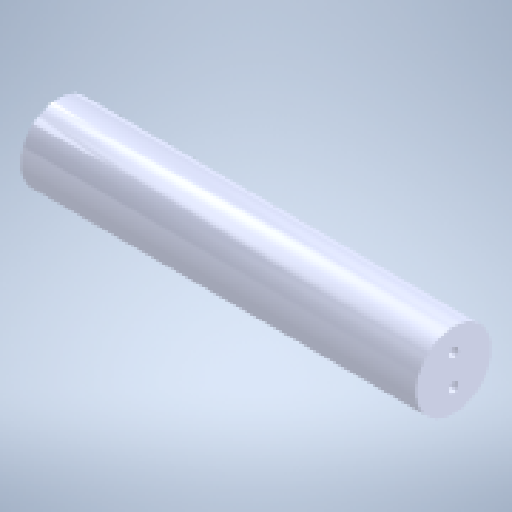
# Autodesk Inventor part: Herramienta Marcador Tubo
Saved by Autodesk Inventor 2023 (Build 270158000, 158)
## iProperties
Created: 2009-11-11
Part Number: Herramienta Marcador Tubo
Material: Generic
Document SubType Name: Modeling
Designer: luisd
Density: 1 g/cm^3
Appearance: Default
Sending System: SolidWorks 2011
Last Author: Antonio
Last Saved: 2012-10-30
SAPModified: X
Author: luisd
Autodesk Inventor part; units mm, degrees
ref_plane "YZ Plane" through (0, 0, 0) normal (1, 0, 0) x (0, 1, 0)
ref_plane "XZ Plane" through (0, 0, 0) normal (0, 1, 0) x (-1, 0, 0)
ref_plane "XY Plane" through (0, 0, 0) normal (0, 0, 1) x (1, 0, 0)
ref_plane "Work Plane1" through (515, 0, 712) normal (1, 0, 0) x (0, 0, -1)
ref_plane "Work Plane2" through (523, 0, 712) normal (1, 0, 0) x (0, 0, -1)
sketch "Sketch2" plane through (523, 0, 712) normal (1, 0, 0) x (0, 0, -1)
  circle A0 centre (0, 0) radius 10
  point P0 (712, 0)
  dimension "d2" = 20
  constraints: 1 centre point
  measures "d2" diameter of A0
extrude "Extrusion2" add sketch "Sketch2" along normal blind 5
sketch "Sketch5" plane through (528, 0, 712) normal (1, 0, 0) x (0, 0, -1)
  circle A0 centre (0, 3.9999) radius 1.25
  circle A1 centre (0, -4.0001) radius 1.25
  point P0 (712, 0)
  point P1 (0, -0.0001)
  dimension "d8" = 2.5
  dimension "d9" = 2.5
  dimension "d13" = 4
  dimension "d14" = 4
  constraints: 2 centre point
  measures "d8" diameter of A0
  measures "d9" diameter of A1
  measures "d13" distance of A0.centre point (0, 0)
  measures "d14" distance of A1.centre point (0, 0)
extrude "Extrusion4" cut sketch "Sketch5" against normal blind 2
sketch "Sketch7" plane through (523, 0, 712) normal (-1, 0, 0) x (0, 0, 1)
  circle A0 centre (0, 0) radius 10 projected
  circle A1 centre (0, 0) radius 8.5
  point P0 (-712, 0)
  dimension "d15" = 17
  constraints: 1 centre point, 1 coincident
  measures "d15" diameter of A1
extrude "Extrusion5" add sketch "Sketch7" along normal blind 100
body "Solid1"
